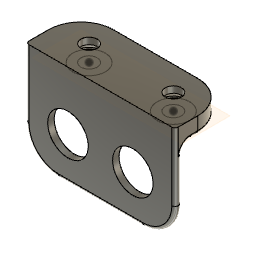
Button Panel v3 (Autodesk Fusion 360 design; units mm, degrees)
Autodesk Fusion 360 part; units mm, degrees
sketch "Sketch1" plane through (0, 0, 0) normal (0, 1, 0) x (1, 0, 0)
  circle A0 centre (-10, 0) radius 6.25
  circle A1 centre (-10, 0) radius 9
  circle A2 centre (10, 0) radius 6.25
  circle A3 centre (10, 0) radius 9
  line L0 (-23, -18) -> (23, -18)
  line L1 (23, -18) -> (23, 3)
  line L2 (13, 13) -> (-13, 13)
  line L3 (-23, 3) -> (-23, -18)
  line L4 (-23, -13) -> (23, -13)
  arc A4 (23, 3) -> (13, 13) centre (13, 3) ccw
  arc A5 (-13, 13) -> (-23, 3) centre (-13, 3) ccw
  dimension "d1" = 12.5
  dimension "d2" = 12.5
  dimension "d3" = 18
  dimension "d4" = 18
  dimension "d5" = 10
  dimension "d6" = 10
  dimension "d7" = 13
  dimension "d9" = 13
  dimension "d10" = 10
  dimension "d11" = 13
  dimension "d12" = 10
  dimension "d13" = 13
  dimension "d14" = 5
  constraint concentric A0 A1
  constraint concentric A2 A3
  constraint horizontal L0
  constraint vertical L1
  constraint horizontal L2
  constraint vertical L3
  constraint coincident L3 L4.start
  constraint coincident L1 L4.end
  constraint perpendicular L1 L4
  constraint tangent L1 A4
  constraint tangent L2 A4
  constraint horizontal origin A2.centre
  constraint horizontal origin A0.centre
  constraint tangent L3 A5
  constraint tangent L2 A5
  measures "d1" diameter of A2
  measures "d2" diameter of A0
  measures "d3" diameter of A1
  measures "d4" diameter of A3
  measures "d5" distance of origin A0.centre
  measures "d6" distance of origin A2.centre
  measures "d7" distance of A2.centre L2
  measures "d9" distance of A2.centre L4
  measures "d10" radius of A4
  measures "d11" distance of A2.centre L1
  measures "d12" radius of A5
  measures "d13" distance of A0.centre L3
  measures "d14" distance of L0 L4
extrude "Extrude1" add sketch "Sketch1" against normal blind 2 contours A1 | A3 | L0 L1 L3 L4 | L1 L2 L3 L4 A4 A5
extrude "Extrude2" add sketch "Sketch1" along normal blind 15 contours L0 L1 L3 L4
sketch "Sketch2" plane through (0, 0, 13) normal (0, 0, -1) x (1, 0, 0)
  line L0 (23, 0) -> (-23, 0)
  line L1 (-23, 0) -> (-23, -15)
  line L2 (-23, -15) -> (23, -15)
  line L3 (23, -15) -> (23, 0)
  circle A0 centre (13, -7.5) radius 2.5
  circle A1 centre (-13, -7.5) radius 2.5
  circle A2 centre (-13, -7.5) radius 5
  circle A3 centre (13, -7.5) radius 5
  dimension "d19" = 5
  dimension "d20" = 5
  dimension "d21" = 10
  dimension "d22" = 10
  dimension "d23" = 7.5
  dimension "d24" = 7.5
  dimension "d25" = 10
  dimension "d26" = 10
  constraint concentric A1 A2
  constraint concentric A0 A3
  measures "d19" diameter of A0
  measures "d20" diameter of A1
  measures "d21" distance of L3 A0.centre
  measures "d22" distance of L1 A1.centre
  measures "d23" distance of L2 A1.centre
  measures "d24" distance of L2 A0.centre
  measures "d25" diameter of A2
  measures "d26" diameter of A3
extrude "Extrude3" cut sketch "Sketch2" against normal up to surface (5 mm away) contours A0 | A1
extrude "Extrude4" cut sketch "Sketch2" against normal up to surface (3 mm away) contours A2 | A3
chamfer "Chamfer1" distance 2.5 angle 45 2 edges at (8.3384, 9.3081, 16) (-17.6616, 9.3081, 16)
fillet "Fillet1" radius 10 2 edges at (23, 15, 15.5) (-23, 15, 15.5)
fillet "Fillet2" radius 3 1 edges at (0, 0, 13)
fillet "Fillet3" radius 1 17 edges at (-23, -2, 7.5) (-20.0711, -2, -10.0711) (0, -2, -13) (20.0711, -2, -10.0711) (23, -2, 7.5) (0, 15, 13) (-20.0711, 12.0711, 13) (-23, 4, 13) (-23, 0.8787, 12.1213) (-23, 0, 3.5) (-20.0711, 0, -10.0711) (0, 0, -13) (20.0711, 0, -10.0711) (23, 0, 3.5) (23, 0.8787, 12.1213) (23, 4, 13) (20.0711, 12.0711, 13)
equation "d1 = d2"
equation "d4 = d3"
equation "d9 = d7"
equation "d11 = d7"
equation "d13 = d7"
equation "d20 = d19"
equation "d22 = d21"
equation "d24 = d23"
equation "d26 = d25"
named bodies: "Button Panel"
